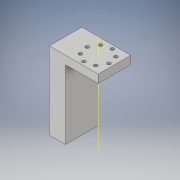
# Autodesk Inventor part: wheel arm stand off
Saved by Autodesk Inventor 2019 (Build 230136000, 136)
## iProperties
Created: 2019-10-26
Part Number: wheel arm stand off
Material: Generic
Document SubType Name: Modeling
Designer: User
Density: 1 g/cm^3
Appearance: Default
Author: User
Autodesk Inventor part; units mm, degrees
ref_plane "YZ Plane" through (0, 0, 0) normal (1, 0, 0) x (0, 1, 0)
ref_plane "XZ Plane" through (0, 0, 0) normal (0, 1, 0) x (-1, 0, 0)
ref_plane "XY Plane" through (0, 0, 0) normal (0, 0, 1) x (1, 0, 0)
sketch "Sketch4" plane through (0, 0, 0) normal (0, 0, 1) x (1, 0, 0)
  line L0 (0, 0) -> (0, 60.2234)
  line L1 (0, 60.2234) -> (25.4, 60.2234)
  line L2 (25.4, 60.2234) -> (25.4, 53.8734)
  line L3 (25.4, 53.8734) -> (0, 53.8734)
  line L4 (0, 60.2234) -> (-12.7, 60.2234)
  line L5 (-12.7, 60.2234) -> (-12.7, 0)
  line L6 (-12.7, 0) -> (0, 0)
  dimension "d25" = 60.2234
  dimension "d26" = 6.35
  dimension "d27" = 25.4
  dimension "d28" = 12.7
  constraints: 14 end point, 5 perpendicular, 1 horizontal, 1 point on line, 1 vertical
  measures "d25" distance of L0.start L0.end
  measures "d26" distance between parallel lines of L1 L3
  measures "d27" distance between parallel lines of L0 L2
  measures "d28" distance of L0.end L4.end
extrude "Extrusion3" add sketch "Sketch4" along normal blind 25.4
sketch "Sketch5" plane through (-12.7, 60.2234, 0) normal (0, 1, 0) x (1, 0, 0)
  line L0 (38.1, 0) -> (38.1, -25.4) projected
  line L1 (38.1, -25.4) -> (0, -25.4) projected
  point P0 (25.4, -12.7)
  point P1 (15.621, -11.3751)
  point P2 (17.5484, -18.678)
  point P3 (24.0751, -22.479)
  point P4 (31.378, -20.5516)
  point P5 (35.179, -14.0249)
  point P6 (33.2516, -6.722)
  point P7 (26.7249, -2.921)
  point P8 (19.422, -4.8484)
  dimension "d36" = 360
  dimension "d45" = 9.779
  dimension "d46" = 12.7
  dimension "d47" = 12.7
  constraints: 9 other
  measures "d45" vertical distance of point (25.4, -12.7) point (26.725, -2.921)
  measures "d46" distance from line of L0 point (25.4, -12.7)
  measures "d47" distance from line of L1 point (25.4, -12.7)
hole "Hole2" at (2.921, 60.2234, 11.3751) at (4.8484, 60.2234, 18.678) at (11.3751, 60.2234, 22.479) at (18.678, 60.2234, 20.5516) at (22.479, 60.2234, 14.0249) at (20.5516, 60.2234, 6.722) at (14.0249, 60.2234, 2.921) at (6.722, 60.2234, 4.8484) direction (0, -1, 0) diameter 2.7178 end through all
body "Solid3"
